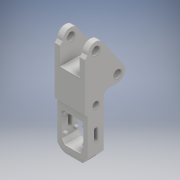
# Autodesk Inventor part: Arm - effector base v2
Saved by Autodesk Inventor 2017 (Build 210142000, 142)
## iProperties
Created: 2016-04-30
Part Number: Arm - effector base v2
Material: Generic
Document SubType Name: Modeling
Designer: Ali
Density: 1 g/cm^3
Appearance: Default
Author: Ali
Autodesk Inventor part; units mm, degrees
ref_plane "YZ Plane" through (0, 0, 0) normal (1, 0, 0) x (0, 1, 0)
ref_plane "XZ Plane" through (0, 0, 0) normal (0, 1, 0) x (-1, 0, 0)
ref_plane "XY Plane" through (0, 0, 0) normal (0, 0, 1) x (1, 0, 0)
sketch "Sketch8" plane through (0, 0, 0) normal (1, 0, 0) x (0, 1, 0)
  circle A0 centre (0, 0) radius 4.5
  circle A1 centre (24.3, -34.6) radius 4.5
  arc A2 (7.3651, 5.1726) -> (-9, 0) centre (0, 0) ccw
  arc A3 (24.3, -43.6) -> (31.6651, -29.4274) centre (24.3, -34.6) ccw
  line L0 (7.3651, 5.1726) -> (31.6651, -29.4274)
  line L1 (24.3, -43.6) -> (9, -43.6)
  line L2 (9, -43.6) -> (9, -103.6)
  line L3 (9, -103.6) -> (-9, -103.6)
  line L4 (-9, -103.6) -> (-9, 0)
  arc A4 (-9, -103.6) -> (9, -103.6) centre (0, -103.6) ccw
  dimension "d64" = 9
  dimension "d65" = 9
  dimension "d66" = 34.6
  dimension "d67" = 24.3
  dimension "d68" = 18
  dimension "d69" = 18
  dimension "d70" = 60
  dimension "d71" = 18
  constraints: 10 end point, 6 point on circle, 5 centre point, 5 tangent, 3 coincident, 1 horizontal, 1 perpendicular, 1 vertical
  measures "d64" diameter of A0
  measures "d65" diameter of A1
  measures "d66" vertical distance of A1.centre point (0, 0)
  measures "d67" horizontal distance of point (0, 0) A1.centre
  measures "d68" diameter of A2
  measures "d69" diameter of A3
  measures "d70" distance of L1.end L2.end
  measures "d71" distance of L2.end L3.end
extrude "Extrusion8" add sketch "Sketch8" along normal blind 6
sketch "Sketch9" plane through (6, 0, 0) normal (1, 0, 0) x (0, 0, -1)
  circle A0 centre (34.6, 24.3) radius 4.5 projected
  line L0 (0, -9) -> (63.6, -9)
  line L1 (43.6, 9) -> (43.6, 24.3) projected
  arc A1 (43.6, 24.3) -> (29.4274, 31.6651) centre (34.6, 24.3) ccw projected
  line L2 (29.4274, 31.6651) -> (-5.1726, 7.3651) projected
  line L3 (23.3108, 9) -> (23.3108, -9)
  line L4 (23.3108, -9) -> (43.6, -9)
  line L5 (43.6, 9) -> (63.6, 9)
  line L6 (63.6, 9) -> (63.6, -9)
  line L7 (63.6, -9) -> (43.6, -9)
  line L8 (99.6, 9) -> (99.6, -9)
  line L9 (99.6, 9) -> (63.6, 9)
  line L10 (63.6, 9) -> (43.6, 9)
  line L11 (63.6, -9) -> (99.6, -9)
  arc A2 (103.6, -9) -> (103.6, 9) centre (103.6, 0) ccw projected
  line L12 (99.6, 9) -> (103.6, 9)
  line L13 (103.6, 9) -> (43.6, 9) projected
  line L14 (103.6, -9) -> (99.6, -9)
  line L15 (0, -9) -> (103.6, -9) projected
  arc A3 (41.1, 24.3) -> (28.3655, 26.1387) centre (34.6, 24.3) ccw
  line L16 (41.1, 24.3) -> (41.1, 9)
  line L17 (41.1, 9) -> (43.6, 9)
  line L18 (28.3655, 26.1387) -> (23.3108, 9)
  point P0 (14.6712, 21.3016)
  point P1 (23.3108, 27.3693)
  dimension "d74" = 20
  dimension "d80" = 36
  dimension "d186" = 2
  constraints: 30 end point, 4 point on circle, 3 collinear, 3 perpendicular, 3 point on line, 1 centre point, 1 horizontal, 1 parallel, 1 tangent, 1 vertical
  measures "d74" distance of L0.end L7.end
  measures "d80" distance between parallel lines of L8 L6
  measures "d186" radial gap between concentric circles of A0 A3
extrude "Extrusion9" add sketch "Sketch9" along normal blind 11 contours L3 L18 A3 L16 L17 L5 L6 L0 | L8 L12 A2 L14
sketch "Sketch11" plane through (6, 0, 0) normal (1, 0, 0) x (0, 0, -1)
  line L0 (63.6, 9) -> (63.6, -9) projected
  line L1 (63.6, -9) -> (99.6, -9) projected
  line L2 (99.6, -9) -> (99.6, 9) projected
  line L3 (99.6, 9) -> (63.6, 9) projected
  point P0 (0, 0)
extrude "Extrusion11" cut sketch "Sketch11" against normal blind 1
sketch "Sketch12" plane through (5, 0, 0) normal (1, 0, 0) x (0, 0, -1)
  line L0 (63.6, -9) -> (63.6, 9) projected
  line L1 (63.6, 9) -> (99.6, 9) projected
  circle A0 centre (72.6, 6) radius 1.95
  circle A1 centre (90.6, 6) radius 1.95
  circle A2 centre (72.6, -6) radius 1.95
  circle A3 centre (90.6, -6) radius 1.95
  point P0 (0, 0)
  dimension "d87" = 3.9
  dimension "d90" = 18
  dimension "d93" = 12
  dimension "d96" = 3
  dimension "d97" = 9
  constraints: 4 centre point, 1 horizontal, 1 vertical, 6 other
  measures "d87" diameter of A0
  measures "d90" distance of A0.centre A1.centre
  measures "d93" distance of A0.centre A2.centre
  measures "d96" distance from line of L1 A0.centre
  measures "d97" distance from line of L0 A0.centre
extrude "Extrusion12" add sketch "Sketch12" along normal blind 3
chamfer "Chamfer5" distance 0.8 angle 45 4 edges at (8, 6, -70.65) (8, 6, -88.65) (8, -6, -88.65) (8, -6, -70.65)
sketch "Sketch13" plane through (5, 0, 0) normal (1, 0, 0) x (0, 0, -1)
  line L0 (63.6, -9) -> (63.6, 9) projected
  line L1 (76.4835, 0) -> (86.7165, 0) construction
  line L2 (76.4835, -2) -> (86.7165, -2)
  line L3 (86.7165, 2) -> (76.4835, 2)
  arc A0 (76.4835, 2) -> (76.4835, -2) centre (76.4835, 0) ccw
  arc A1 (86.7165, -2) -> (86.7165, 2) centre (86.7165, 0) ccw
  line L4 (63.6, -9) -> (63.6, 9) projected
  point P0 (0, 0)
  point P1 (81.6, 0)
  point P2 (63.6, 0)
  dimension "d103" = 4
  dimension "d104" = 18
  constraints: 8 end point, 4 point on circle, 4 tangent, 2 centre point, 2 midpoint, 1 horizontal, 1 parallel, 1 point on line
  measures "d103" diameter of A1
  measures "d104" distance from line of L0 point (81.6, 0)
extrude "Extrusion13" cut sketch "Sketch13" against normal through all
sketch "Sketch14" plane through (0, 0, 0) normal (-1, 0, 0) x (0, 0, 1)
  arc A0 (-76.4835, -2) -> (-76.4835, 2) centre (-76.4835, 0) ccw projected
  line L0 (-52.4835, 0) -> (-66.2095, 0) construction
  point P0 (-105.4194, 0)
  dimension "d107" = 24
  constraints: 2 end point, 2 point on line, 1 horizontal
  measures "d107" distance of A0.centre L0.start
hole "Hole3" at (0, 0, -52.4835) at (0, 0, -105.4194) direction (1, 0, 0) diameter 3.3 end through all counterbore diameter 7 counterbore depth 9
sketch "Sketch15" plane through (17, -9, -63.6) normal (0, 0, -1) x (-1, 0, 0)
  line L0 (0, 18) -> (12, 18) projected
  line L1 (0, 0) -> (0, 18) projected
  line L2 (12, 0) -> (0, 0) projected
  line L3 (12, 0) -> (12, 18) projected
  point P0 (17, 9)
extrude "Extrusion14" add sketch "Sketch15" along normal blind 3.5
chamfer "Chamfer7" distance 1.5 angle 45 1 edges at (5, 0, -67.1)
chamfer "Chamfer8" distance 3.25 distance2 4.5 1 edges at (5, 0, -99.6) measured on face at (5.5, 0, -99.6)
chamfer "Chamfer9" distance 3.5 angle 45 1 edges at (3, 9, -43.6)
ref_plane "Work Plane1" through (8.5, 0, 0) normal (-1, 0, 0) x (0, 0, 1)
sketch "Sketch16" plane through (8.5, 0, 0) normal (-1, 0, 0) x (0, 0, 1)
  circle A0 centre (-34.6, 24.3) radius 4.5 projected
  circle A1 centre (-34.6, 24.3) radius 3.5
  point P0 (0, 0)
  dimension "d129" = 1
  constraints: 1 centre point
  measures "d129" radial gap between concentric circles of A0 A1
extrude "Extrusion15" add sketch "Sketch16" along normal mid plane 9
chamfer "Chamfer10" distance 1 angle 45 4 edges at (4, 27.8, -34.6) (4, 20.8, -34.6) (13, 27.8, -34.6) (13, 20.8, -34.6)
sketch "Sketch17" plane through (0, -9, 0) normal (0, -1, 0) x (1, 0, 0)
  line L0 (17, -23.3108) -> (17, -67.1) projected
  line L1 (6, -23.3108) -> (17, -23.3108) projected
  line L2 (6, 0) -> (6, -23.3108) projected
  line L3 (0, 0) -> (6, 0) projected
  line L4 (0, 0) -> (0, -103.6) projected
  line L5 (17, -59.623) -> (0, -59.623)
  line L6 (0, -103.6) -> (0, -47.1) projected
  point P0 (0, -102.0018)
  constraints: 2 end point, 2 point on line, 1 perpendicular
extrude "Extrusion16" add sketch "Sketch17" along normal blind 3
chamfer "Chamfer11" distance 3 angle 45 2 edges at (8.5, -12, -59.623) (3, -12, 0)
ref_plane "Work Plane2" through (17, 9, -29.3108) normal (0, 1, 0) x (1, 0, 0)
sketch "Sketch25" plane through (17, 9, -29.3108) normal (0, 1, 0) x (1, 0, 0)
  line L0 (21.5052, 66.4542) -> (-21.5052, 66.4542)
  line L1 (-21.5052, 66.4542) -> (0, 90.239)
  line L2 (0, 90.239) -> (21.5052, 66.4542)
  line L3 (21.5052, 66.4542) -> (21.5052, 90.239)
  line L4 (21.5052, 90.239) -> (0, 90.239)
  line L5 (0, 90.239) -> (-21.5052, 90.239)
  line L6 (-21.5052, 90.239) -> (-21.5052, 66.4542)
  line L7 (0, 11.7892) -> (0, 37.7892) projected
  point P0 (-17, -29.3108)
  point P1 (0, 66.4542)
  constraints: 14 end point, 3 point on line, 2 perpendicular, 1 horizontal, 1 midpoint, 1 vertical
extrude "Extrusion24" cut sketch "Sketch25" against normal through all contours L2 L4 L3 | L6 L5 L1
mirror "Mirror2" about plane through (17, 5.5448, -41.6389) normal (1, 0, 0) separate body
sketch "Sketch26" plane through (25, 0, -52.4835) normal (1, 0, 0) x (0, 0, -1)
  circle A0 centre (0, 0) radius 1.65 projected
  line L0 (2.8, -1.6166) -> (0, -3.2332)
  line L1 (0, -3.2332) -> (-2.8, -1.6166)
  line L2 (-2.8, -1.6166) -> (-2.8, 1.6166)
  line L3 (-2.8, 1.6166) -> (0, 3.2332)
  line L4 (0, 3.2332) -> (2.8, 1.6166)
  line L5 (2.8, 1.6166) -> (2.8, -1.6166)
  circle A1 centre (52.9359, 0) radius 1.65 projected
  line L6 (55.7359, -1.6166) -> (52.9359, -3.2332)
  line L7 (52.9359, -3.2332) -> (50.1359, -1.6166)
  line L8 (50.1359, -1.6166) -> (50.1359, 1.6166)
  line L9 (50.1359, 1.6166) -> (52.9359, 3.2332)
  line L10 (52.9359, 3.2332) -> (55.7359, 1.6166)
  line L11 (55.7359, 1.6166) -> (55.7359, -1.6166)
  point P0 (-52.4835, 0)
  dimension "d193" = 5.6
  dimension "d194" = 5.6
  constraints: 24 end point, 2 coincident, 26 other
  measures "d193" distance between parallel lines of L3 L0
  measures "d194" distance between parallel lines of L7 L10
extrude "Extrusion26" cut sketch "Sketch26" against normal blind 3
chamfer "Chamfer16" distance 1.5 angle 45 2 edges at (9, 0, -107.0694) (9, 0, -54.1335)
